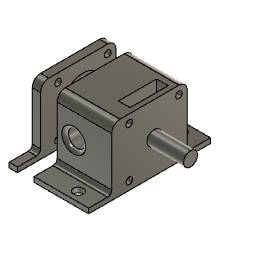
pelletizer_gen1 (Autodesk Fusion 360 design; units mm, degrees)
Autodesk Fusion 360 part; units mm, degrees
note: some values were not read from the file. Set by a fixed rule: which face or edge a step refers to.
sketch "Skizze1" plane through (0, 0, 0) normal (1, 0, 0) x (0, 1, 0)
  circle A0 centre (0, 0) radius 4.25
  circle A1 centre (0, 0) radius 10
  circle A2 centre (40, 0) radius 4
  circle A3 centre (40, 0) radius 11
  circle A4 centre (0, 0) radius 10.25
  line L0 (-12.5, 12.5) -> (12.5, 12.5)
  line L1 (12.5, 12.5) -> (12.5, -12.5)
  line L2 (12.5, -12.5) -> (-12.5, -12.5)
  line L3 (-12.5, -12.5) -> (-12.5, 12.5)
  line L4 (-12.5, 12.5) -> (12.5, -12.5) construction
  line L5 (12.5, 12.5) -> (-12.5, -12.5) construction
  circle A5 centre (0, 0) radius 11
  line L6 (-12.5, 0) -> (-17.5, 0)
  line L7 (-17.5, 0) -> (-17.5, 10)
  line L8 (-17.5, 0) -> (-17.5, -10)
  line L9 (-17.5, -10) -> (-12.5, -10)
  line L10 (-17.5, 10) -> (-12.5, 10)
  line L11 (12.5, 0) -> (-12.5, 0)
  circle A6 centre (0, 0) radius 11.125
  line L12 (0, -12.5) -> (0, -9.5)
  line L13 (0, -8) -> (-9, -8)
  line L14 (-9, -8) -> (-9, -12.5)
  line L15 (0, -8) -> (9, -8)
  line L16 (9, -8) -> (9, -12.5)
  line L17 (9, -12.5) -> (-9, -12.5)
  line L18 (-12.5, 0) -> (-11.125, 0)
  line L19 (-9.3125, 2.5) -> (-14.3125, 2.5)
  line L20 (-14.3125, 2.5) -> (-14.3125, -2.5)
  line L21 (-14.3125, -2.5) -> (-9.3125, -2.5)
  line L22 (-9.3125, -2.5) -> (-9.3125, 2.5)
  line L23 (-9.3125, 2.5) -> (-14.3125, -2.5) construction
  line L24 (-14.3125, 2.5) -> (-9.3125, -2.5) construction
  line L25 (-12.5, -12.5) -> (-27.5, -12.5)
  line L26 (-27.5, -12.5) -> (-27.5, -8.5)
  line L27 (-27.5, -8.5) -> (-12.5, -8.5)
  line L28 (-12.5, -8.5) -> (-12.5, -12.5)
  line L29 (12.5, -12.5) -> (27.5, -12.5)
  line L30 (27.5, -12.5) -> (27.5, -8.5)
  line L31 (27.5, -8.5) -> (12.5, -8.5)
  line L32 (12.5, -8.5) -> (12.5, -12.5)
  line L33 (12.5, -12.5) -> (9.5, -12.5)
  line L34 (9.5, -12.5) -> (9.5, -9.5)
  line L35 (9.5, -9.5) -> (12.5, -9.5)
  line L36 (12.5, -9.5) -> (12.5, -12.5)
  line L37 (-12.5, -12.5) -> (-9.5, -12.5)
  line L38 (-9.5, -12.5) -> (-9.5, -9.5)
  line L39 (-9.5, -9.5) -> (-12.5, -9.5)
  line L40 (-12.5, -9.5) -> (-12.5, -12.5)
  circle A7 centre (9.5, -9.5) radius 1.5
  circle A8 centre (-9.5, -9.5) radius 1.5
  line L41 (-12.5, 12.5) -> (-9.5, 12.5)
  line L42 (-9.5, 12.5) -> (-9.5, 9.5)
  line L43 (-9.5, 9.5) -> (-12.5, 9.5)
  line L44 (-12.5, 9.5) -> (-12.5, 12.5)
  line L45 (12.5, 12.5) -> (9.5, 12.5)
  line L46 (9.5, 12.5) -> (9.5, 9.5)
  line L47 (9.5, 9.5) -> (12.5, 9.5)
  line L48 (12.5, 9.5) -> (12.5, 12.5)
  circle A9 centre (9.5, 9.5) radius 1.5
  circle A10 centre (-9.5, 9.5) radius 1.5
  circle A11 centre (75, 0) radius 12.3
  circle A12 centre (75, 0) radius 10
  line L49 (95, -20) -> (55, -20)
  line L50 (55, -20) -> (55, 20)
  line L51 (55, 20) -> (95, 20)
  line L52 (95, 20) -> (95, -20)
  line L53 (95, -20) -> (55, 20) construction
  line L54 (55, -20) -> (60, -20)
  circle A13 centre (90, -15) radius 2
  circle A14 centre (90, 15) radius 2
  circle A15 centre (60, -15) radius 2
  circle A16 centre (60, 15) radius 2
  line L55 (55, -20) -> (58.5858, -16.4142) construction
  line L56 (60, -15) -> (95, 20) construction
  circle A17 centre (75, 0) radius 11.25
  circle A18 centre (75, 0) radius 4.3
  line L57 (95, -17) -> (95, -20)
  line L58 (55, -20) -> (41, -20)
  line L59 (41, -20) -> (41, -17)
  line L60 (41, -17) -> (55, -17)
  line L61 (55, -17) -> (55, -20)
  line L62 (95, -17) -> (109, -17)
  line L63 (109, -17) -> (109, -20)
  line L64 (109, -20) -> (95, -20)
  point P0 (-11.8125, 0)
  point P1 (75, 0)
  dimension "d1" = 8.5
  dimension "d2" = 20
  dimension "d7" = 8
  dimension "d8" = 22
  dimension "d11" = 20.5
  dimension "d12" = 25
  dimension "d13" = 25
  dimension "d14" = 22
  dimension "d15" = 5
  dimension "d16" = 10
  dimension "d17" = 10
  dimension "d20" = 22.25
  dimension "d36" = 9
  dimension "d40" = 5
  dimension "d61" = 15
  dimension "d62" = 4
  dimension "d63" = 15
  dimension "d64" = 4
  dimension "d87" = 3
  dimension "d88" = 3
  dimension "d89" = 3
  dimension "d90" = 3
  dimension "d91" = 3
  dimension "d92" = 3
  dimension "d93" = 3
  dimension "d94" = 3
  dimension "d95" = 3
  dimension "d96" = 3
  dimension "d97" = 3
  dimension "d98" = 3
  dimension "d116" = 24.6
  dimension "d117" = 20
  dimension "d124" = 5
  dimension "d128" = 4
  dimension "d129" = 4
  dimension "d130" = 4
  dimension "d131" = 4
  dimension "d132" = 22.5
  dimension "d138" = 8.6
  dimension "d153" = 14
  dimension "d154" = 3
  constraint coincident A0.centre A1.centre
  constraint concentric A0 A1
  constraint concentric A2 A3
  constraint concentric A1 A4
  constraint horizontal L0
  constraint perpendicular L0 L1
  constraint parallel L0 L2
  constraint parallel L1 L3
  constraint coincident L4 A0.centre
  constraint coincident L5 A0.centre
  constraint midpoint L3 L6.start
  constraint perpendicular L3 L6
  constraint perpendicular L6 L7
  constraint perpendicular L6 L8
  constraint coincident L3 L9.end
  constraint perpendicular L3 L9
  constraint coincident L3 L10.end
  constraint perpendicular L3 L10
  constraint midpoint L1 L11.start
  constraint concentric A1 A6
  constraint midpoint L2 L12.start
  constraint perpendicular L2 L12
  constraint horizontal L13
  constraint coincident L2 L14.end
  constraint perpendicular L2 L14
  constraint horizontal L15
  constraint coincident L2 L16.end
  constraint perpendicular L2 L16
  constraint coincident L11 L18.end
  constraint coincident A6 L18.end
  constraint horizontal L19
  constraint perpendicular L19 L20
  constraint parallel L19 L21
  constraint parallel L20 L22
  constraint coincident L23 P0
  constraint coincident L24 P0
  constraint midpoint L18 P0
  constraint horizontal L25
  constraint vertical L26
  constraint horizontal L27
  constraint vertical L28
  constraint horizontal L29
  constraint vertical L30
  constraint horizontal L31
  constraint vertical L32
  constraint horizontal L33
  constraint vertical L34
  constraint horizontal L35
  constraint vertical L36
  constraint horizontal L37
  constraint vertical L38
  constraint horizontal L39
  constraint vertical L40
  constraint coincident L34.end L35.start
  constraint coincident L38.end L39.start
  constraint horizontal L41
  constraint vertical L42
  constraint horizontal L43
  constraint vertical L44
  constraint horizontal L45
  constraint vertical L46
  constraint horizontal L47
  constraint vertical L48
  constraint coincident L46.end L47.start
  constraint coincident L42.end L43.start
  constraint concentric A11 A12
  constraint horizontal L49
  constraint perpendicular L49 L50
  constraint parallel L49 L51
  constraint parallel L50 L52
  constraint coincident L53 P1
  constraint coincident P1 L55
  constraint coincident P1 A11.centre
  constraint horizontal L54
  constraint coincident A15.centre L56.start
  constraint coincident A15 L55.end
  constraint collinear L55 L56
  constraint concentric A11 A17
  constraint concentric A17 A18
  constraint vertical L57
  constraint horizontal L58
  constraint vertical L59
  constraint horizontal L60
  constraint vertical L61
  constraint horizontal L62
  constraint vertical L63
  constraint horizontal L64
  measures "d1" diameter of A0
  measures "d2" diameter of A1
  measures "d7" diameter of A2
  measures "d8" diameter of A3
  measures "d11" diameter of A4
  measures "d12" distance of L1.end L2.end
  measures "d13" distance of L0.end L1.end
  measures "d14" diameter of A5
  measures "d15" distance of L6.start L6.end
  measures "d16" distance of L6.end L7.end
  measures "d17" distance of L6.end L8.end
  measures "d20" diameter of A6
  measures "d36" distance of L13.start L15.end
  measures "d40" distance of L20.end L21.end
  measures "d61" distance of L2.end L25.end
  measures "d62" distance of L2.end L27.end
  measures "d63" distance of L1.end L29.end
  measures "d64" distance of L1.end L31.end
  measures "d87" distance of L1.end L33.end
  measures "d88" distance of L1.end L35.end
  measures "d89" distance of L2.end L37.end
  measures "d90" distance of L2.end L39.end
  measures "d91" diameter of A7
  measures "d92" diameter of A8
  measures "d93" distance of L0.start L41.end
  measures "d94" distance of L0.start L43.end
  measures "d95" distance of L0.end L45.end
  measures "d96" distance of L0.end L47.end
  measures "d97" diameter of A9
  measures "d98" diameter of A10
  measures "d116" diameter of A11
  measures "d117" diameter of A12
  measures "d124" distance of L49.end L54.end
  measures "d128" diameter of A13
  measures "d129" diameter of A14
  measures "d130" diameter of A15
  measures "d131" diameter of A16
  measures "d132" diameter of A17
  measures "d138" diameter of A18
  measures "d153" distance of L49.end L58.end
  measures "d154" distance of L49.end L60.end
extrude "Extrusion1" add sketch "Skizze1" along normal blind 32 contours A0 L11 | A0 L11 makes body 1
extrude "Extrusion2" add sketch "Skizze1" against normal blind 20 separate body contours A0 A1 L11 L13 L15 L21 L22 | A0 A1 L11 L19 L22 | A1 L11 L21 L22 | A1 L11 L19 L22 | A1 L13 L15 makes body 2
combine "Kombinieren1" operation add target body 1 tool bodies 2
extrude "Extrusion3" add sketch "Skizze1" along normal blind 7 separate body contours A3 makes body 3
move_body "Verschieben1" bodies 3 to x (1, 0, 0) y (0, 1, 0) z (0, 0, 1) at (2, 0, 0)
move_body "Verschieben2" bodies 3 to x (1, 0, 0) y (0, 1, 0) z (0, 0, 1) at (0, -40, 0)
copy_body "Körper kopieren/einfügen1" bodies 3 makes body 4
move_body "Verschieben3" bodies 4 to x (1, 0, 0) y (0, 1, 0) z (0, 0, 1) at (23, 0, 0)
move_body "Verschieben4" bodies 4 to x (1, 0, 0) y (0, 1, 0) z (0, 0, 1) at (-12, 0, 0)
extrude "Extrusion4" add sketch "Skizze1" against normal blind 21 separate body contours A5 L11 A6 L15 | A5 L11 A6 L19 | A5 L11 A6 L19 | A5 A6 L12 L15 | L0 L1 L3 L11 A6 L19 L42 L43 L46 L47 A9 A10 | L1 L11 A6 L15 L16 L32 L35 A7 | A5 L11 A6 L21 | L3 L11 A6 L18 L19 | A5 A6 L12 L13 | L2 A6 L12 L15 L16 L17 A7 | A5 A6 L13 L21 | L3 L11 A6 L18 L21 | L2 A6 L12 L13 L14 L17 A8 | L0 L1 L45 L46 L47 L48 A9 | L3 A6 L13 L14 L21 L28 L39 A8 | L0 L3 L41 L42 L43 L44 A10 | L16 L34 L35 A7 | L16 A7 | L46 L47 A9 | L46 L47 A9 | L1 L2 L32 L33 L34 L35 L36 A7 | L42 L43 A10 | L42 L43 A10 | L2 L16 L34 A7 | L2 L14 L38 A8 | L34 L35 A7 | L14 A8 | L14 L38 L39 A8 | L2 L3 L28 L37 L38 L39 L40 A8 | L38 L39 A8 makes body 5
extrude "Extrusion5" add sketch "Skizze1" along normal blind 24 contours L1 L11 A6 L15 L16 L32 L35 A7 | L2 A6 L12 L15 L16 L17 A7 | L3 L11 A6 L18 L21 | L2 A6 L12 L13 L14 L17 A8 | L3 A6 L13 L14 L21 L28 L39 A8 | L16 L34 L35 A7 | L16 A7 | L1 L2 L32 L33 L34 L35 L36 A7 | L2 L16 L34 A7 | L2 L14 L38 A8 | L34 L35 A7 | L14 A8 | L14 L38 L39 A8 | L2 L3 L28 L37 L38 L39 L40 A8 | L38 L39 A8 bodies 5
extrude "Extrusion6" add sketch "Skizze1" along normal blind 3.5 from surface at 9.25 separate body contours A0 A1 L11 L13 L15 L21 L22 | A0 A1 L11 L19 L22 | A1 A4 L11 L15 | A1 A4 L11 L19 | A1 L11 L21 L22 | A1 L11 L19 L22 | A1 A4 L11 L19 | A1 A4 L12 L15 | A1 L13 L15 | A4 A5 L11 L15 | A4 A5 L11 L19 | A1 A4 L11 L21 | A4 A5 L11 L19 | A1 A4 L12 L13 | A4 A5 L12 L15 | A5 L11 A6 L15 | A5 L11 A6 L19 | A1 A4 L13 L21 | A4 A5 L11 L21 | A5 L11 A6 L19 | A4 A5 L12 L13 | A5 A6 L12 L15 | A4 A5 L13 L21 | A5 L11 A6 L21 | A5 A6 L12 L13 | A5 A6 L13 L21 makes body 6
copy_body "Körper kopieren/einfügen2" bodies 6 makes body 7
move_body "Verschieben5" bodies 7 to x (1, 0, 0) y (0, 1, 0) z (0, 0, 1) at (11, 0, 0)
combine "Kombinieren2" operation add target body 7 tool bodies 5
combine "Kombinieren3" operation add target body 6 tool bodies 7
extrude "Extrusion7" add sketch "Skizze1" along normal blind 1.5 separate body contours A0 A1 L11 L13 L15 L21 L22 | A0 A1 L11 L19 L22 | A1 A4 L11 L15 | A1 A4 L11 L19 | A1 L11 L21 L22 | A1 L11 L19 L22 | A1 A4 L11 L19 | A1 A4 L12 L15 | A1 L13 L15 | A4 A5 L11 L15 | A4 A5 L11 L19 | A1 A4 L11 L21 | A4 A5 L11 L19 | A1 A4 L12 L13 | A4 A5 L12 L15 | A5 L11 A6 L15 | A5 L11 A6 L19 | A1 A4 L13 L21 | A4 A5 L11 L21 | A5 L11 A6 L19 | A4 A5 L12 L13 | A5 A6 L12 L15 | A4 A5 L13 L21 | A5 L11 A6 L21 | A5 A6 L12 L13 | A5 A6 L13 L21 makes body 8
combine "Kombinieren4" operation add target body 8 tool bodies 6
fillet "Abrundung1" radius 1 1 edges at (0, 0, 11.125) on bodies 8
extrude "Extrusion8" cut 1 faces at (24, -11.8769, -5.2597) along direction (-1, 0, 0) blind 0.25 on bodies 8 bodies 8
fillet "Abrundung2" radius 5 1 edges at (-10.5, -12.5, 12.5) on bodies 8
fillet "Abrundung3" radius 5 1 edges at (-10.5, 12.5, 12.5) on bodies 8
extrude "Extrusion9" cut sketch "Skizze1" against normal blind 15 from surface at -3 contours A1 A4 L12 L15 | A1 L13 L15 | A1 A4 L12 L13 | A4 A5 L12 L15 | A4 A5 L12 L13 | A5 A6 L12 L15 | A5 A6 L12 L13 | L2 A6 L12 L15 L16 L17 A7 | L2 A6 L12 L13 L14 L17 A8 | L16 A7 | L14 A8 bodies 8
extrude "Extrusion10" add sketch "Skizze1" against normal blind 21 contours L3 L6 L7 L10 L19 L20 L44 | L3 L6 L19 L20 | L3 L6 L20 L21 | L3 L6 L8 L20 L21 L27 | L3 L8 L9 L27 L28 L40 bodies 8
extrude "Extrusion11" cut 1 faces at (-7, -15.8333, 10) along direction (0, 0, -1) blind 2.5 on bodies 8 bodies 8
extrude "Extrusion12" add 1 faces at (-7, -15.8333, -10) along direction (0, 0, -1) blind 2.5 on bodies 8 bodies 8
hole "Bohrung2" at (-11, -17.5, 0) direction (0, 1, 0) diameter 10.4 depth 10 tip angle 118 bodies 8
extrude "Extrusion13" add 1 faces at (-10.6667, -17.5, -10.0667) along direction (0, -1, 0) blind 4 on bodies 8 bodies 8
extrude "Extrusion14" add 1 faces at (-8, 8.0332, -8) along direction (0, 0, -1) blind 4.5 on bodies 8 bodies 8
extrude "Extrusion15" add 1 faces at (-8, -8.0332, -8) along direction (0, 0, -1) blind 4.5 on bodies 8 bodies 8
extrude "Extrusion16" add sketch "Skizze1" along normal blind 23.75 contours L1 L29 L30 L31 L32 L36 | L3 L8 L9 L27 L28 L40 | L3 L8 L9 L25 L26 L27 L28 L40 bodies 8
hole "Bohrung3" at (6.35, -20, -8.5) direction (0, 0, -1) diameter 5 depth 9 tip angle 118 bodies 8
hole "Bohrung4" at (18.75, -20, -8.5) direction (0, 0, -1) diameter 5 depth 9 tip angle 118 bodies 8
hole "Bohrung5" at (5, 20, -8.5) direction (0, 0, -1) diameter 5 depth 9 tip angle 118 bodies 8
hole "Bohrung6" at (18.75, 20, -8.5) direction (0, 0, -1) diameter 5 depth 9 tip angle 118 bodies 8
extrude "Extrusion17" cut sketch "Skizze1" against normal blind 15 from surface at -6 contours L16 L34 L35 A7 | L16 A7 | L46 L47 A9 | L46 L47 A9 | L42 L43 A10 | L42 L43 A10 | L34 L35 A7 | L14 A8 | L14 L38 L39 A8 | L38 L39 A8 bodies 8
fillet "Abrundung4" radius 2.5 2 edges at (11.875, 27.5, -8.5) (11.875, -27.5, -8.5) on bodies 8
extrude "Extrusion18" cut 4 faces at (-6, -10.4271, 9.3931) (-6, 8.5729, 9.3931) (-6, -10.0991, -9.0435) (-6, 8.9009, -9.0435) along direction (1, 0, 0) blind 95 on bodies 8 bodies 8
extrude "Extrusion19" cut 1 faces at (23.75, 0.1059, -8.0408) along direction (-1, 0, 0) blind 11 on bodies 8 bodies 8
extrude "Extrusion20" add 1 faces at (-21, -17.959, -2.2132) along direction (-1, 0, 0) blind 2 on bodies 8 bodies 8
extrude "Extrusion21" add sketch "Skizze1" along normal blind 3 separate body contours A0 L11 | A0 A1 L11 L13 L15 L21 L22 | A0 A1 L11 L19 L22 | A0 L11 | A1 A4 L11 L15 | A1 A4 L11 L19 | A1 L11 L21 L22 | A1 L11 L19 L22 | A1 A4 L11 L19 | A1 A4 L12 L15 | A1 L13 L15 | A4 A5 L11 L15 | A4 A5 L11 L19 | A1 A4 L11 L21 | A4 A5 L11 L19 | A1 A4 L12 L13 | A4 A5 L12 L15 | A5 L11 A6 L15 | A5 L11 A6 L19 | A1 A4 L13 L21 | A4 A5 L11 L21 | A5 L11 A6 L19 | A4 A5 L12 L13 | A5 A6 L12 L15 | L0 L1 L3 L11 A6 L19 L42 L43 L46 L47 A9 A10 | L1 L11 A6 L15 L16 L32 L35 A7 | A4 A5 L13 L21 | A5 L11 A6 L21 | L3 L11 A6 L18 L19 | A5 A6 L12 L13 | L2 A6 L12 L15 L16 L17 A7 | A5 A6 L13 L21 | L3 L11 A6 L18 L21 | L2 A6 L12 L13 L14 L17 A8 | L0 L1 L45 L46 L47 L48 A9 | L3 A6 L13 L14 L21 L28 L39 A8 | L0 L3 L41 L42 L43 L44 A10 | L1 L2 L32 L33 L34 L35 L36 A7 | L2 L16 L34 A7 | L2 L14 L38 A8 | L2 L3 L28 L37 L38 L39 L40 A8 makes body 9
move_body "Verschieben6" bodies 9 to x (1, 0, 0) y (0, 1, 0) z (0, 0, 1) at (-35, 0, 0)
fillet "Abrundung5" radius 5 2 edges at (-33.5, -12.5, 12.5) (-33.5, 12.5, 12.5) on bodies 9
extrude "Extrusion22" add 1 faces at (-11.3333, -21.5, -10.0667) along direction (0, -1, 0) blind 3 on bodies 8 bodies 8
move_body "Verschieben7" bodies 9 to x (1, 0, 0) y (0, 1, 0) z (0, 0, 1) at (-10, 0, 0)
extrude "Extrusion23" add sketch "Skizze1" along normal blind 20 separate body contours A11 | A17 makes body 10
move_body "Verschieben8" bodies 1 to x (1, 0, 0) y (0, 1, 0) z (0, 0, 1) at (0, 30, 0)
move_body "Ausrichten1" bodies 1 to x (1, 0, 0) y (0, 1, 0) z (0, 0, 1) at (20, 45, 0)
move_body "Verschieben9" bodies 3 to x (1, 0, 0) y (0, 1, 0) z (0, 0, 1) at (0, 25, 0)
move_body "Ausrichten2" bodies 3 to x (1, 0, 0) y (0, 1, 0) z (0, 0, 1) at (43, 50, 0)
move_body "Verschieben10" bodies 3 to x (1, 0, 0) y (0, 1, 0) z (0, 0, 1) at (-20, 0, 0)
move_body "Verschieben11" bodies 3 to x (1, 0, 0) y (0, 1, 0) z (0, 0, 1) at (-5, 0, 0)
extrude "Extrusion24" add sketch "Skizze1" along normal blind 30 separate body contours L49 L50 L51 L52 L54 L57 L61 makes body 11
extrude "Extrusion25" add sketch "Skizze1" along normal blind 10 from surface at 20 contours A11 bodies 11
extrude "Extrusion26" add sketch "Skizze1" along normal blind 3 from surface at 27 contours A11 | A12 | A17 bodies 11
sketch "Skizze2" plane through (0, 0, -20) normal (0, 0, -1) x (1, 0, 0)
  line L0 (0, -55) -> (0, -95)
  line L1 (0, -95) -> (30, -95)
  line L2 (30, -95) -> (30, -55)
  line L3 (30, -55) -> (0, -55)
  line L4 (27.0024, -75, -20) -> (20, -75, -20)
  line L5 (20, -86.25) -> (20, -63.75)
  line L6 (27, -63.75) -> (27, -86.25)
  line L7 (27, -86.25) -> (20, -63.75) construction
  line L8 (20, -86.25) -> (27, -63.75) construction
  line L9 (0, -75) -> (12, -75)
  line L10 (12, -75) -> (12, -78)
  line L11 (12, -78) -> (0, -78)
  line L12 (12, -75) -> (12, -72)
  line L13 (12, -72) -> (0, -72)
  line L14 (0, -72) -> (0, -78)
  line L15 (0, -78) -> (12, -78)
  line L16 (12, -78) -> (12, -72)
  line L17 (12, -72) -> (0, -72)
  line L18 (0, -72) -> (0, -78)
  line L19 (20, -75) -> (20, -63.5)
  line L20 (20, -75) -> (20, -86.5)
  line L21 (27, -86.25) -> (27, -86.5)
  line L22 (27, -86.5) -> (20, -86.5)
  line L23 (27, -63.75) -> (27, -63.5)
  line L24 (27, -63.5) -> (20, -63.5)
  point P0 (23.5, -75)
  dimension "d142" = 22.5
  dimension "d168" = 12
  dimension "d169" = 3
  dimension "d170" = 3
  dimension "d207" = 11.5
  dimension "d208" = 11.5
  dimension "d209" = 0.25
  dimension "d210" = 0.25
  constraint parallel L5 L6
  constraint coincident L7 P0
  constraint coincident L8 P0
  constraint midpoint L0 L9.start
  constraint perpendicular L0 L9
  constraint perpendicular L9 L10
  constraint coincident L0 L11.end
  constraint perpendicular L0 L11
  constraint perpendicular L9 L12
  constraint coincident L0 L13.end
  constraint perpendicular L0 L13
  constraint horizontal L15
  constraint vertical L16
  constraint horizontal L17
  constraint vertical L18
  constraint midpoint L5 L19.start
  constraint perpendicular L1 L20
  constraint perpendicular L20 L22
  constraint perpendicular L19 L24
  measures "d142" distance of L5.start L5.end
  measures "d168" distance of L9.start L9.end
  measures "d169" distance of L9.end L10.end
  measures "d170" distance of L9.end L12.end
  measures "d207" distance of L19.start L19.end
  measures "d208" distance of L19.start L20.end
  measures "d209" distance of L6.end L21.end
  measures "d210" distance of L6.start L23.end
extrude "Extrusion27" cut sketch "Skizze2" against normal blind 25 from surface at -18 contours L5 L6 L19 L20 L21 L22 L23 L24 bodies 3 11
extrude "Extrusion28" add sketch "Skizze1" against normal blind 3 contours L49 L50 L51 L52 L54 L57 L61 bodies 11
extrude "Extrusion29" add sketch "Skizze1" along normal blind 3 from surface at 17 contours A11 | A12 | A17 bodies 3 11
extrude "Extrusion30" add sketch "Skizze1" along normal blind 30 contours L52 L57 L62 L63 L64 | L50 L58 L59 L60 L61 bodies 3
extrude "Extrusion31" add sketch "Skizze1" against normal blind 3 contours L52 L57 L62 L63 L64 | L50 L58 L59 L60 L61 bodies 3
move_body "Verschieben12" bodies 4 to x (1, 0, 0) y (0, 1, 0) z (0, 0, 1) at (7, 75, 0)
combine "Kombinieren5" operation cut target body 3 tool bodies 4 keep tools
move_body "Verschieben13" bodies 4 to x (1, 0, 0) y (0, 1, 0) z (0, 0, 1) at (0, -57, 0)
extrude "Extrusion33" add 1 faces at (24.6667, 63.6431, -2) along direction (0, 0, 1) blind 22 on bodies 3 bodies 3
extrude "Extrusion34" add 1 faces at (24.6667, 86.3569, -2) along direction (0, 0, 1) blind 22 on bodies 3 bodies 3
extrude "Extrusion35" cut sketch "Skizze2" against normal blind 14 contours L0 L9 L12 L13 L14 L16 L17 L18 | L0 L9 L10 L11 L14 L15 L16 L18 bodies 3
hole "Bohrung7" at (7, 55, 0) direction (0, 1, 0) diameter 10.4 depth 9 tip angle 118 bodies 3
extrude "Extrusion36" add 1 faces at (24.0618, 55, 1.1295) along direction (0, -1, 0) blind 0.5 on bodies 3 bodies 3
extrude "Extrusion37" add 1 faces at (24.0618, 54.5, 1.1295) along direction (0, -1, 0) blind 5.05 on bodies 3 bodies 3
extrude "Extrusion38" add 1 faces at (8, 41, -18) along direction (0, -1, 0) blind 5 on bodies 3 bodies 3
extrude "Extrusion39" add 1 faces at (8, 36, -18) along direction (0, -1, 0) blind 0.55 on bodies 3 bodies 3
fillet "Abrundung8" radius 5 2 edges at (13.5, 49.45, 20) (13.5, 95, 20) on bodies 3
fillet "Abrundung9" radius 2.5 2 edges at (13.5, 49.45, -17) (13.5, 95, -17) on bodies 3
hole "Bohrung8" at (18, 41.2, -17) direction (0, 0, -1) diameter 6 depth 10 tip angle 118 bodies 3
hole "Bohrung9" at (18, 103.425, -17) direction (0, 0, -1) diameter 6 depth 10 tip angle 118 bodies 3
extrude "Extrusion40" cut 1 faces at (24.6667, 86.0708, 9.1199) along direction (0, 1, 0) blind 0.15 on bodies 3 bodies 3
extrude "Extrusion41" cut 1 faces at (24.6667, 63.9292, 9.1199) along direction (0, -1, 0) blind 0.15 on bodies 3 bodies 3
extrude "Extrusion42" cut sketch "Skizze1" along normal blind 7 from surface at 20 contours A12 | A17 bodies 3
extrude "Extrusion43" cut sketch "Skizze2" against normal blind 20 from surface at -20 contours L5 L6 L19 L20 L21 L22 L23 L24 bodies 3
fillet "Abrundung10" radius 2 1 edges at (8.8804, 49.45, 4.8481) on bodies 3
extrude "Extrusion44" add 1 faces at (-3, 53.8667, 0.1667) along direction (-1, 0, 0) blind 5 from surface at 10 on bodies 3 bodies 3 makes body 12
extrude "Extrusion45" add sketch "Skizze1" against normal blind 3 from surface at -15 contours A11 | A12 | A17 | A18 bodies 12
extrude "Extrusion32" [suppressed]
hidden bodies 4 8 9
named bodies: "Fräser", "Kugellager_1", "Kugellager", "Kugellager_2", "Gehause", "Deckel", "Rundrohr", "Gehäuse_Rndrohr", "Deckel_Neu"
